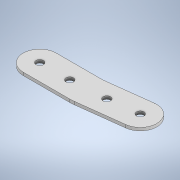
# Autodesk Inventor part: angle bracket
Saved by Autodesk Inventor 2021 (Build 250183000, 183)
## iProperties
Created: 2021-03-09
Part Number: angle bracket
Material: Generic
Document SubType Name: Modeling
Designer: Ferdinand Hubbard
Density: 1 g/cm^3
Appearance: Default
Author: Ferdinand Hubbard
Autodesk Inventor part; units mm, degrees
ref_plane "YZ Plane" through (0, 0, 0) normal (1, 0, 0) x (0, 1, 0)
ref_plane "XZ Plane" through (0, 0, 0) normal (0, 1, 0) x (-1, 0, 0)
ref_plane "XY Plane" through (0, 0, 0) normal (0, 0, 1) x (1, 0, 0)
sketch "Sketch1" plane through (0, 0, 0) normal (0, 1, 0) x (-1, 0, 0)
  line L0 (-11, 0) -> (-42, 0)
  line L1 (-42, 0) -> (-42, -22) construction
  line L2 (-42, -22) -> (-11, -22)
  line L3 (0, -11) -> (0, -11)
  arc A0 (-42, 0) -> (-44.6811, -0.164) centre (-42, -22) ccw
  line L4 (-42, -22) -> (-44.6811, -0.164) construction
  line L5 (-42, -22) -> (-20, -22) construction
  line L6 (-42, -22) -> (-44.6811, -0.164) construction
  line L7 (-44.6811, -0.164) -> (-75.4501, -3.9419)
  line L8 (-85.0275, -16.2005) -> (-85.0275, -16.2005)
  line L9 (-72.7689, -25.7779) -> (-42, -22)
  line L10 (0, 0) -> (-11, 0) construction
  line L11 (-11, 0) -> (-31, 0) construction
  line L12 (-11, 0) -> (-11, -11) construction
  line L13 (-31, 0) -> (-31, -11) construction
  circle A1 centre (-11, -11) radius 2.5
  circle A2 centre (-31, -11) radius 2.5
  line L14 (-44.6811, -0.164) -> (-55.5991, -1.5045) construction
  line L15 (-55.5991, -1.5045) -> (-54.2586, -12.4226) construction
  line L16 (-54.2586, -12.4226) -> (-74.1095, -14.8599) construction
  circle A3 centre (-74.1095, -14.8599) radius 2.5
  circle A4 centre (-54.2586, -12.4226) radius 2.5
  arc A5 (-11, -22) -> (0, -11) centre (-11, -11) ccw
  arc A6 (0, -11) -> (-11, 0) centre (-11, -11) ccw
  arc A7 (-85.0275, -16.2005) -> (-72.7689, -25.7779) centre (-74.1095, -14.8599) ccw
  arc A8 (-75.4501, -3.9419) -> (-85.0275, -16.2005) centre (-74.1095, -14.8599) ccw
  point P0 (0, -22)
  point P1 (-86.3681, -5.2825)
  point P2 (-83.6869, -27.1185)
  dimension "d0" = 42
  dimension "d3" = 97
  dimension "d4" = 42
  dimension "d5" = 11
  dimension "d6" = 20
  dimension "d7" = 22
  dimension "d8" = 11
  dimension "d9" = 11
  dimension "d10" = 5
  dimension "d11" = 5
  dimension "d12" = 11
  dimension "d13" = 11
  dimension "d14" = 90
  dimension "d15" = 20
  dimension "d16" = 5
  dimension "d17" = 5
  dimension "d20" = 11
  dimension "d21" = 11
  constraints: 34 end point, 11 point on line, 10 point on circle, 9 centre point, 8 tangent, 5 coincident, 5 parallel, 4 perpendicular, 2 equal radius, 2 horizontal, 1 collinear, 1 equal length, 1 vertical
  measures "d0" distance of point (0, -22) L1.end
  measures "d3" angle of L5 L4
  measures "d4" distance of L4.end point (-86.368, -5.282)
  measures "d5" distance of L10.start L10.end
  measures "d6" distance of L10.end L11.end
  measures "d7" distance of point (0, -22) L10.start
  measures "d8" distance of L10.end L12.end
  measures "d9" distance of L11.end L13.end
  measures "d10" diameter of A1
  measures "d11" diameter of A2
  measures "d12" distance of L4.end L14.end
  measures "d13" distance of L14.end L15.end
  measures "d14" angle of L15 L14
  measures "d15" distance of L15.end L16.end
  measures "d16" diameter of A3
  measures "d17" diameter of A4
  measures "d20" radius of A5
  measures "d21" radius of A6
extrude "Extrusion1" add sketch "Sketch1" along normal blind 2
body "Solid1"
